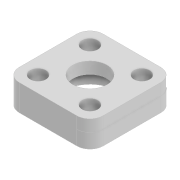
# Autodesk Inventor part: Part16
Saved by Autodesk Inventor 2020.5 (Build 245400000, 400)
## iProperties
Created: 2022-11-15
Part Number: Part16
Material: 一般
Document SubType Name: Modeling
Designer: Administrator
Density: 1 g/cm^3
Appearance: 既定
Author: Administrator
Autodesk Inventor part; units mm, degrees
ref_plane "YZ Plane" through (0, 0, 0) normal (1, 0, 0) x (0, 1, 0)
ref_plane "XZ Plane" through (0, 0, 0) normal (0, 1, 0) x (-1, 0, 0)
ref_plane "XY Plane" through (0, 0, 0) normal (0, 0, 1) x (1, 0, 0)
sketch "スケッチ1" plane through (0, 0, 0) normal (0, 1, 0) x (-1, 0, 0)
  circle A0 centre (0.0113, -0.5464) radius 9.75
  circle A1 centre (0.0113, -0.5464) radius 5
  circle A2 centre (0.0113, -0.5464) radius 5
  circle A3 centre (0.0113, -0.5464) radius 14
  circle A4 centre (-9.8882, 9.3531) radius 1.5
  circle A5 centre (9.9108, -10.4458) radius 1.5
  line L0 (0.0113, -0.5464) -> (9.9108, 9.3531)
  line L1 (0.0113, -0.5464) -> (14.0113, -0.5464) construction
  line L2 (0.0113, -0.5464) -> (-9.8882, 9.3531)
  line L3 (0.0113, -0.5464) -> (14.0113, -0.5464) construction
  line L4 (0.0113, -0.5464) -> (-9.8882, -10.4458)
  line L5 (0.0113, -0.5464) -> (14.0113, -0.5464) construction
  line L6 (0.0113, -0.5464) -> (9.9108, -10.4458)
  line L7 (0.0113, -0.5464) -> (14.0113, -0.5464) construction
  circle A6 centre (9.9108, 9.3531) radius 1.5
  circle A7 centre (-9.8882, -10.4458) radius 1.5
  circle A8 centre (-9.8882, 9.3531) radius 3
  circle A9 centre (9.9108, 9.3531) radius 3
  circle A10 centre (9.9108, -10.4458) radius 3
  circle A11 centre (-9.8882, -10.4458) radius 3
  circle A12 centre (0.0113, -0.5464) radius 6.5
  line L8 (-15.9887, 15.4536) -> (16.0113, 15.4536)
  line L9 (16.0113, 15.4536) -> (16.0113, -16.5464)
  line L10 (16.0113, -16.5464) -> (-15.9887, -16.5464)
  line L11 (-15.9887, -16.5464) -> (-15.9887, 15.4536)
  line L12 (-15.9887, 15.4536) -> (16.0113, -16.5464) construction
  line L13 (16.0113, 15.4536) -> (-15.9887, -16.5464) construction
  circle A13 centre (0.0113, -0.5464) radius 5
  circle A14 centre (0.0113, -0.5464) radius 9.75
  point P0 (0, 0)
  point P1 (0, 0)
  dimension "d0" = 28
  dimension "d1" = 3
  dimension "d2" = 3
  dimension "d3" = 45
  dimension "d4" = 135
  dimension "d5" = 135
  dimension "d6" = 45
  dimension "d7" = 3
  dimension "d8" = 3
  dimension "d9" = 6
  dimension "d10" = 6
  dimension "d11" = 6
  dimension "d12" = 6
  dimension "d13" = 13
  dimension "d14" = 32
  dimension "d15" = 32
  dimension "d18" = 19.5
  constraints: 28 end point, 15 centre point, 10 coincident, 5 horizontal, 4 equal length, 4 point on circle, 2 concentric, 2 midpoint, 2 parallel, 1 perpendicular
  measures "d0" diameter of A3
  measures "d1" diameter of A4
  measures "d2" diameter of A5
  measures "d3" angle of L1 L0
  measures "d4" angle of L3 L2
  measures "d5" angle of L4 L5
  measures "d6" angle of L6 L7
  measures "d7" diameter of A6
  measures "d8" diameter of A7
  measures "d9" diameter of A8
  measures "d10" diameter of A9
  measures "d11" diameter of A10
  measures "d12" diameter of A11
  measures "d13" diameter of A12
  measures "d14" distance of L9.end L10.end
  measures "d15" distance of L8.end L9.end
  measures "d18" diameter of A0
extrude "押し出し1" add sketch "スケッチ1" along normal blind 4.5 contours A0 L6 A12 L0 | A0 L0 A9 A3 A10 L6 | L0 A12 L2 A0 | A0 L2 A8 A3 A9 L0 | L6 A10 A3 A11 L4 A0 | A0 L4 A12 L6 | L2 A12 L4 A0 | A0 L4 A11 A3 A8 L2 | L8 L9 L10 L11
sketch "スケッチ2" plane through (0, 0, 0) normal (0, -1, 0) x (1, 0, 0)
  circle A0 centre (0.0113, -0.5464) radius 9.75
  circle A1 centre (0.0113, -0.5464) radius 5
  circle A2 centre (0.0113, -0.5464) radius 5
  circle A3 centre (0.0113, -0.5464) radius 14
  circle A4 centre (-9.8882, 9.3531) radius 1.5
  circle A5 centre (9.9108, -10.4458) radius 1.5
  line L0 (0.0113, -0.5464) -> (9.9108, 9.3531)
  line L1 (0.0113, -0.5464) -> (14.0113, -0.5464) construction
  line L2 (0.0113, -0.5464) -> (-9.8882, 9.3531)
  line L3 (0.0113, -0.5464) -> (14.0113, -0.5464) construction
  line L4 (0.0113, -0.5464) -> (-9.8882, -10.4458)
  line L5 (0.0113, -0.5464) -> (14.0113, -0.5464) construction
  line L6 (0.0113, -0.5464) -> (9.9108, -10.4458)
  line L7 (0.0113, -0.5464) -> (14.0113, -0.5464) construction
  circle A6 centre (9.9108, 9.3531) radius 1.5
  circle A7 centre (-9.8882, -10.4458) radius 1.5
  circle A8 centre (-9.8882, 9.3531) radius 3
  circle A9 centre (9.9108, 9.3531) radius 3
  circle A10 centre (9.9108, -10.4458) radius 3
  circle A11 centre (-9.8882, -10.4458) radius 3
  circle A12 centre (0.0113, -0.5464) radius 6.5
  line L8 (-15.9887, 15.4536) -> (16.0113, 15.4536)
  line L9 (16.0113, 15.4536) -> (16.0113, -16.5464)
  line L10 (16.0113, -16.5464) -> (-15.9887, -16.5464)
  line L11 (-15.9887, -16.5464) -> (-15.9887, 15.4536)
  line L12 (-15.9887, 15.4536) -> (16.0113, -16.5464) construction
  line L13 (16.0113, 15.4536) -> (-15.9887, -16.5464) construction
  circle A13 centre (0.0113, -0.5464) radius 5
  circle A14 centre (0.0113, -0.5464) radius 9.75
  point P0 (0, 0)
  point P1 (0, 0)
  point P2 (0, 0)
  dimension "d19" = 28
  dimension "d20" = 3
  dimension "d21" = 3
  dimension "d22" = 45
  dimension "d23" = 135
  dimension "d24" = 135
  dimension "d25" = 45
  dimension "d26" = 3
  dimension "d27" = 3
  dimension "d28" = 6
  dimension "d29" = 6
  dimension "d30" = 6
  dimension "d31" = 6
  dimension "d32" = 13
  dimension "d33" = 32
  dimension "d34" = 32
  dimension "d35" = 19.5
  constraints: 28 end point, 15 centre point, 10 coincident, 5 horizontal, 4 equal length, 4 point on circle, 2 concentric, 2 midpoint, 2 parallel, 1 perpendicular
  measures "d19" diameter of A3
  measures "d20" diameter of A4
  measures "d21" diameter of A5
  measures "d22" angle of L1 L0
  measures "d23" angle of L3 L2
  measures "d24" angle of L4 L5
  measures "d25" angle of L6 L7
  measures "d26" diameter of A6
  measures "d27" diameter of A7
  measures "d28" diameter of A8
  measures "d29" diameter of A9
  measures "d30" diameter of A10
  measures "d31" diameter of A11
  measures "d32" diameter of A12
  measures "d33" distance of L9.end L10.end
  measures "d34" distance of L8.end L9.end
  measures "d35" diameter of A0
extrude "押し出し2" add sketch "スケッチ2" along normal blind 5.5 contours A0 L0 A9 A3 A10 L6 | A0 L2 A8 A3 A9 L0 | L6 A10 A3 A11 L4 A0 | A0 L4 A11 A3 A8 L2 | A9 A3 A6 L0 | L0 A6 A3 A9 | A10 A3 A5 L6 | L6 A5 A3 A10 | A8 A3 A4 L2 | L2 A4 A3 A8 | A9 A3 A6 | A11 A3 A7 L4 | L4 A7 A3 A11 | A10 A3 A5 | A8 A3 A4 | A3 A7 A11 | L8 L9 L10 L11
fillet "フィレット1" radius 5 7 edges at (16.0113, -2.75, -16.5464) (15.9887, 2.25, -16.5464) (16.0113, -2.75, 15.4536) (15.9887, 2.25, 15.4536) (-16.0113, 2.25, 15.4536) (-15.9887, -2.75, -16.5464) (-16.0113, 2.25, -16.5464)
